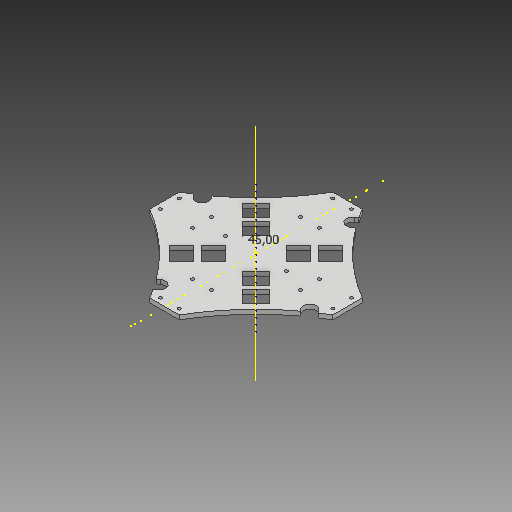
# Autodesk Inventor part: grundplatte_oben
Saved by Autodesk Inventor 2019 (Build 230136000, 136)
## iProperties
Created: 2018-07-23
Part Number: grundplatte_oben
Material: Generisch
Document SubType Name: Modeling
Designer: juliu
Density: 1 g/cm^3
Appearance: Vorgabe
Author: juliu
Autodesk Inventor part; units mm, degrees
ref_plane "YZ Plane" through (0, 0, 0) normal (1, 0, 0) x (0, 1, 0)
ref_plane "XZ Plane" through (0, 0, 0) normal (0, 1, 0) x (-1, 0, 0)
ref_plane "XY Plane" through (0, 0, 0) normal (0, 0, 1) x (1, 0, 0)
sketch "Skizze2" plane through (0, 0, 0) normal (0, 0, 1) x (1, 0, 0)
  line L0 (-13.75, 85) -> (13.75, 85)
  arc A0 (13.75, 85) -> (85, 13.75) centre (186.2357, 186.2357) ccw
  line L1 (-260.73, 0) -> (260.73, 0) projected
  line L2 (0, -260.73) -> (0, 260.73) projected
  line L3 (-85, 13.75) -> (-85, -13.75)
  line L4 (-13.75, -85) -> (13.75, -85)
  line L5 (85, 13.75) -> (85, -13.75)
  arc A1 (85, -13.75) -> (13.75, -85) centre (186.2357, -186.2357) ccw
  arc A2 (-13.75, -85) -> (-85, -13.75) centre (-186.2357, -186.2357) ccw
  arc A3 (-85, 13.75) -> (-13.75, 85) centre (-186.2357, 186.2357) ccw
  point P0 (0, 0)
  dimension "d26" = 360
  dimension "d11" = 27.5
  dimension "d13" = 200
  dimension "d16" = 13.75
  dimension "d17" = 85
  dimension "d18" = 85
  constraints: 8 end point, 8 point on circle, 6 symmetric about line, 4 centre point, 2 equal radius, 2 horizontal, 2 vertical, 1 parallel
  measures "d11" distance of L0.start L0.end
  measures "d13" radius of A0
  measures "d16" distance from line of L1 L5.start
  measures "d17" distance from line of L2 L5.start
  measures "d18" distance between parallel lines of L1 L0
extrude "Extrusion1" add sketch "Skizze2" along normal blind 4
sketch "Skizze3" plane through (0, 0, 4) normal (0, 0, 1) x (1, 0, 0)
  line L0 (13.75, 85) -> (-13.75, 85) projected
  line L1 (0, -119) -> (0, 119) projected
  point P0 (0, 0)
  point P1 (-8.75, 80)
  point P2 (-8.75, 50)
  point P3 (8.75, 80)
  point P4 (8.75, 50)
  point P5 (-80, 8.75)
  point P6 (-80, -8.75)
  point P7 (-50, -8.75)
  point P8 (-50, 8.75)
  point P9 (0, 0)
  point P10 (-8.75, -80)
  point P11 (8.75, -80)
  point P12 (8.75, -50)
  point P13 (-8.75, -50)
  point P14 (0, 0)
  point P15 (80, -8.75)
  point P16 (80, 8.75)
  point P17 (50, 8.75)
  point P18 (50, -8.75)
  point P19 (0, 0)
  dimension "d21" = 5
  dimension "d22" = 30
  dimension "d26" = 360
  dimension "d35" = 17.5
  constraints: 2 coincident, 2 symmetric about line, 1 vertical alignment, 19 other
  measures "d21" distance from line of L0 point (-8.75, 80)
  measures "d22" distance of point (-8.75, 80) point (-8.75, 50)
  measures "d35" distance of point (8.75, 50) point (-8.75, 50)
hole "Bohrung1" at (-8.75, 80, 4) at (-8.75, 50, 4) at (8.75, 80, 4) at (8.75, 50, 4) at (-80, 8.75, 4) at (-80, -8.75, 4) at (-50, -8.75, 4) at (-50, 8.75, 4) at (-8.75, -80, 4) at (8.75, -80, 4) at (8.75, -50, 4) at (-8.75, -50, 4) at (80, -8.75, 4) at (80, 8.75, 4) at (50, 8.75, 4) at (50, -8.75, 4) direction (0, 0, -1) diameter 3 end through all
sketch "Skizze4" plane through (0, 0, 4) normal (0, 0, 1) x (1, 0, 0)
  line L0 (-119, 0) -> (119, 0) projected
  line L1 (0, -119) -> (0, 119) projected
  line L2 (-70.7107, 0) -> (0, 70.7107)
  line L3 (70.7107, 0) -> (0, 70.7107)
  line L4 (70.7107, 0) -> (0, -70.7107)
  line L5 (0, -70.7107) -> (-70.7107, 0)
  line L6 (-70.7107, 0) -> (0, -70.7107)
  line L7 (55.4416, -27.1574) -> (17.3594, 10.9249)
  point P0 (0, 0)
  point P1 (28.2843, 0)
  point P2 (-28.2843, 0)
  dimension "d26" = 360
  dimension "d40" = 100
  dimension "d41" = 45
  dimension "d42" = 30
  dimension "d43" = 30
  constraints: 12 end point, 7 point on line, 2 perpendicular, 1 collinear, 1 parallel
  measures "d40" distance of L3.start L2.end
  measures "d41" angle of L0 L3
  measures "d42" distance from line of L4 point (28.284, 0)
  measures "d43" distance from line of L2 point (-28.284, 0)
hole "Bohrung2" at (28.2843, 0, 4) at (-28.2843, 0, 4) direction (0, 0, -1) diameter 3 end through all
sketch "Skizze5" plane through (0, 0, 4) normal (0, 0, 1) x (1, 0, 0)
  line L0 (-61.0486, 61.0486) -> (63.6647, -63.6647)
  line L1 (0, -119) -> (0, 119) projected
  point P0 (0, 0)
  dimension "d26" = 360
  dimension "d51" = 45
  constraints: 2 end point, 1 point on line
  measures "d51" angle of L0 L1
sketch "Skizze6" plane through (0, 0, 4) normal (0, 0, 1) x (1, 0, 0)
  line L0 (19.0919, -31.8198) -> (7.7782, -20.5061)
  line L1 (7.7782, -20.5061) -> (20.5061, -7.7782)
  line L2 (20.5061, -7.7782) -> (31.8198, -19.0919)
  line L3 (31.8198, -19.0919) -> (19.0919, -31.8198)
  line L4 (-119, 119) -> (119, -119) projected
  line L5 (22.6274, -35.3553) -> (33.9411, -46.669)
  line L6 (33.9411, -46.669) -> (46.669, -33.9411)
  line L7 (46.669, -33.9411) -> (35.3553, -22.6274)
  line L8 (35.3553, -22.6274) -> (22.6274, -35.3553)
  point P0 (0, 0)
  dimension "d26" = 360
  dimension "d52" = 16
  dimension "d53" = 18
  dimension "d54" = 20
  dimension "d55" = 18
  dimension "d56" = 16
  dimension "d57" = 5
  constraints: 16 end point, 4 perpendicular, 2 parallel, 2 other
  measures "d52" distance of L1.end L2.end
  measures "d53" distance of L0.end L1.end
  measures "d54" distance from line of point (0, 0) L1
  measures "d55" distance of L5.end L6.end
  measures "d56" distance of L6.end L7.end
  measures "d57" distance between parallel lines of L3 L8
extrude "Extrusion2" cut sketch "Skizze6" against normal blind 10
pattern_circular "Runde Anordnung1" count 4 over 360 about axis through (0, 0, -10) along (0, 0, 1) of "Extrusion2"
sketch "Skizze7" plane through (0, 0, 4) normal (0, 0, 1) x (1, 0, 0)
  line L0 (-119, 0) -> (119, 0) projected
  line L1 (0, -119) -> (0, 119) projected
  arc A0 (13.75, 85) -> (85, 13.75) centre (186.2357, 186.2357) ccw projected
  line L2 (-7.6995, 95.7117) -> (21.2973, 109.2466)
  line L3 (14.7698, 66.3429) -> (38.9042, 83.2183)
  arc A1 (16.5618, 74.9172) -> (23.4382, 65.0828) centre (20, 70) ccw
  line L4 (20, 70) -> (23.4382, 65.0828) construction
  line L5 (20, 70) -> (16.5618, 74.9172) construction
  line L6 (16.5618, 74.9172) -> (18.9651, 76.5976)
  line L7 (23.4382, 65.0828) -> (25.8415, 66.7632)
  line L8 (25.8415, 66.7632) -> (18.9651, 76.5976)
  point P0 (0, 0)
  dimension "d26" = 360
  dimension "d63" = 70
  dimension "d64" = 20
  dimension "d66" = 180
  dimension "d67" = 12
  constraints: 14 end point, 4 point on circle, 2 line through centre, 2 parallel, 2 point on line, 2 tangent, 1 centre point, 1 coincident
  measures "d63" distance from line of L0 point (20, 70)
  measures "d64" distance from line of L1 point (20, 70)
  measures "d66" angle of L4 L5
  measures "d67" distance of L7.end L6.end
extrude "Extrusion3" cut sketch "Skizze7" against normal blind 10 fills toward (15.1238, 66.5904) open curves A1
pattern_circular "Runde Anordnung2" count 4 over 360 about axis through (0, 0, -10) along (0, 0, 1) of "Extrusion3"
